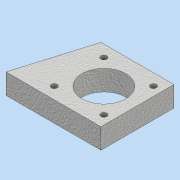
# Autodesk Inventor part: Wspornik łożyska osi Y - prawa strona
Saved by Autodesk Inventor 2018 (Build 220112000, 112)
## iProperties
Created: 2019-01-27
Part Number: Wspornik łożyska osi Y - prawa strona
Material: Ogólny
Document SubType Name: Modeling
Designer: Dawid
Density: 1 g/cm^3
Appearance: Aluminium odlewane
Author: Dawid
Autodesk Inventor part; units mm, degrees
ref_plane "YZ Plane" through (0, 0, 0) normal (1, 0, 0) x (0, 1, 0)
ref_plane "XZ Plane" through (0, 0, 0) normal (0, 1, 0) x (-1, 0, 0)
ref_plane "XY Plane" through (0, 0, 0) normal (0, 0, 1) x (1, 0, 0)
sketch "Szkic6" plane through (0, 0, 0) normal (0, 0, 1) x (1, 0, 0)
  circle A0 centre (-40, -42) radius 2
  circle A1 centre (-40, -8) radius 2
  circle A2 centre (-6, -8) radius 2
  circle A3 centre (-6, -42) radius 2
  circle A4 centre (-23, -25) radius 15
  line L0 (0, -50) -> (0, 0)
  line L1 (-50, 0) -> (0, 0)
  line L2 (-65, -50) -> (-50, 0)
  line L3 (-23, -25) -> (-23, -50)
  line L4 (-23, -50) -> (0, -50)
  line L5 (-23, -50) -> (-65, -50)
  dimension "d30" = 25
  constraints: 12 end point, 5 centre point, 2 perpendicular
  measures "d30" distance of L3.start L3.end
extrude "Wyciągnięcie proste4" add sketch "Szkic6" along normal blind 14
